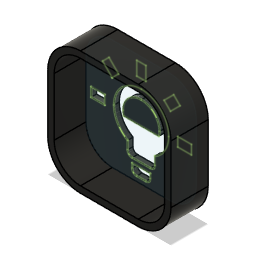
Trellis Keycap lightbulb on 50 (Autodesk Fusion 360 design; units mm, degrees)
Autodesk Fusion 360 part; units mm, degrees
sketch "Sketch1" plane through (0, 0, 0) normal (0, 0, 1) x (1, 0, 0)
  line L0 (2.72, 5) -> (-2.72, 5)
  line L1 (-5, 2.72) -> (-5, -2.72)
  line L2 (-2.72, -5) -> (2.72, -5)
  line L3 (5, -2.72) -> (5, 2.72)
  line L4 (5, 5) -> (-5, -5) construction
  line L5 (-5, 5) -> (5, -5) construction
  arc A0 (5, 2.72) -> (2.72, 5) centre (2.72, 2.72) ccw
  arc A1 (2.72, -5) -> (5, -2.72) centre (2.72, -2.72) ccw
  arc A2 (-5, -2.72) -> (-2.72, -5) centre (-2.72, -2.72) ccw
  arc A3 (-2.72, 5) -> (-5, 2.72) centre (-2.72, 2.72) ccw
  line L6 (-2.72, -5.2) -> (2.72, -5.2)
  arc A4 (2.72, -5.2) -> (5.2, -2.72) centre (2.72, -2.72) ccw
  line L7 (5.2, -2.72) -> (5.2, 2.72)
  arc A5 (5.2, 2.72) -> (2.72, 5.2) centre (2.72, 2.72) ccw
  line L8 (2.72, 5.2) -> (-2.72, 5.2)
  arc A6 (-2.72, 5.2) -> (-5.2, 2.72) centre (-2.72, 2.72) ccw
  line L9 (-5.2, 2.72) -> (-5.2, -2.72)
  arc A7 (-5.2, -2.72) -> (-2.72, -5.2) centre (-2.72, -2.72) ccw
  line L10 (-2.72, -5.8) -> (2.72, -5.8)
  arc A8 (2.72, -5.8) -> (5.8, -2.72) centre (2.72, -2.72) ccw
  line L11 (5.8, -2.72) -> (5.8, 2.72)
  arc A9 (5.8, 2.72) -> (2.72, 5.8) centre (2.72, 2.72) ccw
  line L12 (2.72, 5.8) -> (-2.72, 5.8)
  arc A10 (-2.72, 5.8) -> (-5.8, 2.72) centre (-2.72, 2.72) ccw
  line L13 (-5.8, 2.72) -> (-5.8, -2.72)
  arc A11 (-5.8, -2.72) -> (-2.72, -5.8) centre (-2.72, -2.72) ccw
  dimension "d1" = 10
  dimension "d2" = 10
  dimension "d3" = 2.28
  dimension "d4" = 0.2
  dimension "d5" = 0.8
  constraint horizontal L0
  constraint perpendicular L0 L1
  constraint parallel L0 L2
  constraint parallel L1 L3
  constraint coincident L4 origin
  constraint coincident L5 origin
  constraint coincident L4.start L0
  constraint coincident L4.start L3
  constraint tangent L0 A0
  constraint tangent L3 A0
  constraint coincident L5.end L3
  constraint coincident L5.end L2
  constraint tangent L3 A1
  constraint tangent L2 A1
  constraint equal A0 A1
  constraint coincident L4.end L2
  constraint coincident L4.end L1
  constraint tangent L2 A2
  constraint tangent L1 A2
  constraint equal A0 A2
  constraint coincident L5.start L1
  constraint coincident L5.start L0
  constraint tangent L1 A3
  constraint tangent L0 A3
  constraint equal A0 A3
  measures "d1" distance of L4.end L5.end
  measures "d2" distance of L5.start L4.end
  measures "d3" radius of A0
extrude "Extrude1" add sketch "Sketch1" along normal blind 3 contours L10 A8 L11 A9 L12 A10 L13 A11 makes body 1
extrude "Extrude2" add sketch "Sketch1" against normal blind 0.5 contours L0 L1 L2 L3 A0 A1 A2 A3 | L6 A4 L7 A5 L8 A6 L9 A7 | L10 A8 L11 A9 L12 A10 L13 A11 bodies 1
sketch "Sketch2" plane through (0, 0, 0) normal (0, 0, 1) x (1, 0, 0)
  line L0 (-2.72, -5.2) -> (2.72, -5.2)
  arc A0 (2.72, -5.2) -> (5.2, -2.72) centre (2.72, -2.72) ccw
  line L1 (5.2, -2.72) -> (5.2, 2.72)
  arc A1 (5.2, 2.72) -> (2.72, 5.2) centre (2.72, 2.72) ccw
  line L2 (2.72, 5.2) -> (-2.72, 5.2)
  arc A2 (-2.72, 5.2) -> (-5.2, 2.72) centre (-2.72, 2.72) ccw
  line L3 (-5.2, 2.72) -> (-5.2, -2.72)
  arc A3 (-5.2, -2.72) -> (-2.72, -5.2) centre (-2.72, -2.72) ccw
  line L4 (-4.7048, 0.4027) -> (-3.4185, 0.4027)
  line L5 (-3.4185, 0.4027) -> (-3.4185, -0.4548)
  line L6 (-3.4185, -0.4548) -> (-4.7048, -0.4548)
  line L7 (-4.7048, -0.4548) -> (-4.7048, 0.4027)
  spline S0 degree 3 poles (-0.8458, -4.3139) (-0.8458, -4.5712) (-0.6743, -4.7427) (-0.417, -4.7427) knots 0 0 0 0 1 1 1 1
  line L8 (-0.417, -4.7427) -> (0.4406, -4.7427)
  spline S1 degree 3 poles (0.4406, -4.7427) (0.6978, -4.7427) (0.8694, -4.5712) (0.8694, -4.3139) knots 0 0 0 0 1 1 1 1
  line L9 (0.8694, -4.3139) -> (0.8694, -3.8851)
  line L10 (0.8694, -3.8851) -> (-0.8458, -3.8851)
  line L11 (-0.8458, -3.8851) -> (-0.8458, -4.3139)
  line L12 (0.4406, 4.6906) -> (-0.417, 4.6906)
  line L13 (-0.417, 4.6906) -> (-0.417, 3.4042)
  line L14 (-0.417, 3.4042) -> (0.4406, 3.4042)
  line L15 (0.4406, 3.4042) -> (0.4406, 4.6906)
  line L16 (-3.0326, 3.6186) -> (-3.6329, 3.0183)
  line L17 (-3.6329, 3.0183) -> (-2.7324, 2.1179)
  line L18 (-2.7324, 2.1179) -> (-2.1321, 2.7182)
  line L19 (-2.1321, 2.7182) -> (-3.0326, 3.6186)
  line L20 (3.4421, 0.4027) -> (3.4421, -0.4548)
  line L21 (3.4421, -0.4548) -> (4.7284, -0.4548)
  line L22 (4.7284, -0.4548) -> (4.7284, 0.4027)
  line L23 (4.7284, 0.4027) -> (3.4421, 0.4027)
  line L24 (3.0562, 3.6186) -> (2.1557, 2.7182)
  line L25 (2.1557, 2.7182) -> (2.756, 2.1179)
  line L26 (2.756, 2.1179) -> (3.6564, 3.0183)
  line L27 (3.6564, 3.0183) -> (3.0562, 3.6186)
  spline S2 degree 3 poles (2.5845, -0.026) (2.5845, -0.9694) (2.0699, -1.8269) (1.2981, -2.2557) knots 0 0 0 0 1 1 1 1
  line L28 (1.2981, -2.2557) -> (1.2981, -3.0275)
  spline S3 degree 3 poles (1.2981, -3.0275) (1.2981, -3.2848) (1.1266, -3.4563) (0.8694, -3.4563) knots 0 0 0 0 1 1 1 1
  line L29 (0.8694, -3.4563) -> (-0.8458, -3.4563)
  spline S4 degree 3 poles (-0.8458, -3.4563) (-1.1031, -3.4563) (-1.2746, -3.2848) (-1.2746, -3.0275) knots 0 0 0 0 1 1 1 1
  line L30 (-1.2746, -3.0275) -> (-1.2746, -2.2557)
  spline S5 degree 3 poles (-1.2746, -2.2557) (-2.0464, -1.8269) (-2.5609, -0.9694) (-2.5609, -0.026) knots 0 0 0 0 1 1 1 1
  spline S6 degree 3 poles (-2.5609, -0.026) (-2.5609, 1.3889) (-1.4032, 2.5467) (0.0118, 2.5467) knots 0 0 0 0 1 1 1 1
  spline S7 degree 3 poles (0.0118, 2.5467) (1.4268, 2.5467) (2.5845, 1.3889) (2.5845, -0.026) knots 0 0 0 0 1 1 1 1
  spline S8 degree 3 poles (-1.7033, -0.026) (-1.7033, -0.1761) (-1.6819, -0.3176) (-1.6433, -0.4548) knots 0 0 0 0 1 1 1 1
  line L31 (-1.6433, -0.4548) -> (1.6669, -0.4548)
  spline S9 degree 3 poles (1.6669, -0.4548) (1.7055, -0.3176) (1.7269, -0.1761) (1.7269, -0.026) knots 0 0 0 0 1 1 1 1
  spline S10 degree 3 poles (1.7269, -0.026) (1.7269, 0.9216) (0.9594, 1.6891) (0.0118, 1.6891) knots 0 0 0 0 1 1 1 1
  spline S11 degree 3 poles (0.0118, 1.6891) (-0.9358, 1.6891) (-1.7033, 0.9216) (-1.7033, -0.026) knots 0 0 0 0 1 1 1 1
extrude "Extrude3" cut sketch "Sketch2" against normal blind 0.5 contours L4 L5 L6 L7 | S0 L8 S1 L9 L10 L11 | L12 L13 L14 L15 | L16 L17 L18 L19 | L20 L21 L22 L23 | L24 L25 L26 L27 | S2 L28 S3 L29 S4 L30 S5 S6 S7 bodies 1 makes body 2 at (0.0118, 0.2598, -0.5)
extrude "Extrude4" add sketch "Sketch2" against normal blind 0.5 separate body contours L4 L5 L6 L7 | S0 L8 S1 L9 L10 L11 | L12 L13 L14 L15 | L16 L17 L18 L19 | L20 L21 L22 L23 | L24 L25 L26 L27 | S2 L28 S3 L29 S4 L30 S5 S6 S7 makes body 3 at (3.8708, 0.1169, 0) makes body 4 at (-4.2761, 0.1169, 0) makes body 5 at (2.8561, 2.6181, 0) makes body 6 at (-0.417, -1.0551, 0) makes body 7 at (-2.6324, 2.8182, 0) makes body 8 at (-0.1311, 3.833, 0) makes body 9 at (-0.1311, -4.171, 0)
named bodies: "Keycap", "Keycap (1)"
